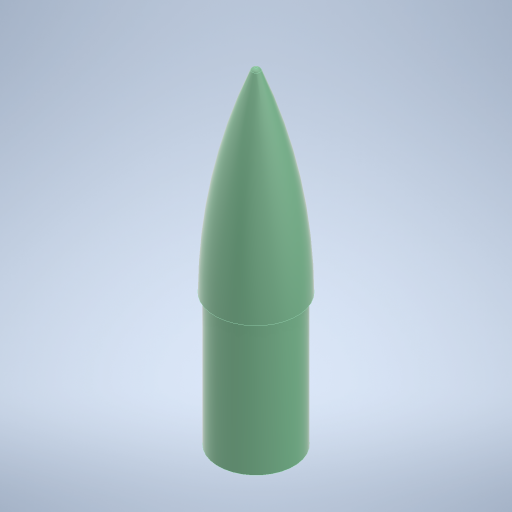
# Autodesk Inventor part: nose-cone
Saved by Autodesk Inventor 2023.2 (Build 272271000, 271)
## iProperties
Created: 2022-12-17
Part Number: nose-cone
Material: Papier
Document SubType Name: Modeling
Designer: jacob
Density: 0.68 g/cm^3
Appearance: Gładki — ciemna zieleń morska
Author: jacob
Autodesk Inventor part; units mm, degrees
ref_plane "YZ Plane" through (0, 0, 0) normal (1, 0, 0) x (0, 1, 0)
ref_plane "XZ Plane" through (0, 0, 0) normal (0, 1, 0) x (-1, 0, 0)
ref_plane "XY Plane" through (0, 0, 0) normal (0, 0, 1) x (1, 0, 0)
sketch "Szkic1" plane through (0, 0, 0) normal (0, 0, 1) x (1, 0, 0)
  line L0 (0, 0) -> (-22.98, 0)
  line L1 (-2.0098, 198) -> (0, 198)
  line L2 (0, 198) -> (0, 0)
  line L3 (-22.98, 0) -> (-22.98, 80)
  line L4 (-22.98, 80) -> (-25, 80)
  arc A0 (-2.0098, 198) -> (-25, 80) centre (296.3098, 78.6381) ccw
  dimension "d0" = 22.98
  dimension "d10" = 80
  dimension "d11" = 198
  dimension "d13" = 2.02
  constraints: 10 end point, 3 horizontal, 2 point on circle, 1 centre point, 1 perpendicular, 1 vertical
  measures "d0" distance of L0.start L0.end
  measures "d10" distance of L0.end L3.end
  measures "d11" vertical distance of L0.end L1.start
  measures "d13" distance of L3.end L4.end
revolve "Obrót1" add sketch "Szkic1" angle 360 about axis through (0, 198, 0) along (0, -1, 0)
fillet "Zaokrąglenie2" radius 2 1 edges at (2.0098, 198, 0)
sketch "Szkic4" plane through (0, 0, 0) normal (0, -1, 0) x (1, 0, 0)
  circle A0 centre (0, 0) radius 22.98 projected
  circle A1 centre (0, 0) radius 22.98 projected
  circle A2 centre (0, 0) radius 22.5
  point P0 (0, 0)
  dimension "d21" = 0.48
  dimension "d22" = 45
  constraints: 1 centre point
  measures "d21" radial gap between concentric circles of A0 A2
  measures "d22" diameter of A2
extrude "parachute" cut sketch "Szkic4" against normal blind 100 contours A2
